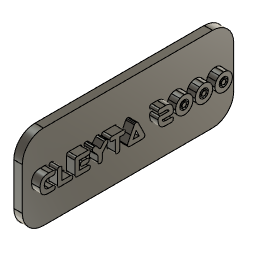
cleyta - placa v2 (Autodesk Fusion 360 design; units mm, degrees)
Autodesk Fusion 360 part; units mm, degrees
note: some values were not read from the file. Chosen so that the rebuilt part matches the saved one: which face or edge a step refers to.
(part 1 of 2)
sketch "Sketch1" plane through (0, 0, 0) normal (1, 0, 0) x (0, 1, 0)
  line L0 (-62.7452, 16.4403) -> (-22.7452, 16.4403)
  line L1 (-17.7452, 11.4403) -> (-17.7452, 1.4403)
  line L2 (-22.7452, -3.5597) -> (-62.7452, -3.5597)
  line L3 (-67.7452, 1.4403) -> (-67.7452, 11.4403)
  arc A0 (-62.7452, 16.4403) -> (-67.7452, 11.4403) centre (-62.7452, 11.4403) ccw
  arc A1 (-17.7452, 11.4403) -> (-22.7452, 16.4403) centre (-22.7452, 11.4403) ccw
  arc A2 (-22.7452, -3.5597) -> (-17.7452, 1.4403) centre (-22.7452, 1.4403) ccw
  arc A3 (-67.7452, 1.4403) -> (-62.7452, -3.5597) centre (-62.7452, 1.4403) ccw
  point P0 (-67.7452, 16.4403)
  point P1 (-17.7452, 16.4403)
  point P2 (-67.7452, -3.5597)
  dimension "d1" = 50
  dimension "d2" = 20
  dimension "d3" = 5
  constraint horizontal L0
  constraint vertical L1
  constraint horizontal L2
  constraint vertical L3
  constraint coincident P0 L0
  constraint coincident P0 L3
  constraint tangent L0 A0
  constraint tangent L3 A0
  constraint coincident P1 L0
  constraint coincident P1 L1
  constraint tangent L0 A1
  constraint tangent L1 A1
  constraint equal A0 A1
  constraint tangent L1 A2
  constraint tangent L2 A2
  constraint equal A0 A2
  constraint coincident P2 L2
  constraint coincident P2 L3
  constraint tangent L2 A3
  constraint tangent L3 A3
  constraint equal A0 A3
  measures "d1" distance of P0 P1
  measures "d2" distance of P0 P2
  measures "d3" radius of A0
extrude "Extrude1" add sketch "Sketch1" along normal blind 5
sketch "Sketch2" plane through (5, 0, 0) normal (1, 0, 0) x (0, 1, 0)
  arc A0 (-62.7452, 16.4403) -> (-67.7452, 11.4403) centre (-62.7452, 11.4403) ccw
  line L0 (-67.7452, 11.4403) -> (-67.7452, 1.4403)
  arc A1 (-67.7452, 1.4403) -> (-62.7452, -3.5597) centre (-62.7452, 1.4403) ccw
  line L1 (-62.7452, -3.5597) -> (-22.7452, -3.5597)
  arc A2 (-22.7452, -3.5597) -> (-17.7452, 1.4403) centre (-22.7452, 1.4403) ccw
  line L2 (-17.7452, 1.4403) -> (-17.7452, 11.4403)
  arc A3 (-17.7452, 11.4403) -> (-22.7452, 16.4403) centre (-22.7452, 11.4403) ccw
  line L3 (-22.7452, 16.4403) -> (-62.7452, 16.4403)
  line L4 (-62.4235, 8.5936) -> (-61.4376, 8.5911)
  spline S0 degree 3 poles (-61.4376, 8.5911) (-61.1111, 8.5861) (-60.9466, 8.4234) (-60.9447, 8.1031) knots 0 0 0 0 1 1 1 1
  spline S1 degree 3 poles (-60.9447, 8.1031) (-60.9466, 7.771) (-61.1117, 7.6058) (-61.4401, 7.6077) knots 0 0 0 0 1 1 1 1
  line L5 (-61.4401, 7.6077) -> (-62.421, 7.6052)
  spline S2 degree 3 poles (-62.421, 7.6052) (-63.0766, 7.6102) (-63.4044, 7.283) (-63.4044, 6.6243) knots 0 0 0 0 1 1 1 1
  spline S3 degree 3 poles (-63.4044, 6.6243) (-63.4044, 5.97) (-63.0766, 5.6415) (-62.421, 5.6384) knots 0 0 0 0 1 1 1 1
  line L6 (-62.421, 5.6384) -> (-61.4401, 5.6384)
  spline S4 degree 3 poles (-61.4401, 5.6384) (-61.1117, 5.6315) (-60.9472, 5.4689) (-60.9472, 5.1505) knots 0 0 0 0 1 1 1 1
  spline S5 degree 3 poles (-60.9472, 5.1505) (-60.9472, 4.8214) (-61.1098, 4.6563) (-61.4351, 4.655) knots 0 0 0 0 1 1 1 1
  line L7 (-61.4351, 4.655) -> (-62.421, 4.655)
  spline S6 degree 3 poles (-62.421, 4.655) (-63.7341, 4.655) (-64.3915, 5.3119) (-64.3928, 6.6268) knots 0 0 0 0 1 1 1 1
  spline S7 degree 3 poles (-64.3928, 6.6268) (-64.3928, 7.9392) (-63.7366, 8.5948) (-62.4235, 8.5936) knots 0 0 0 0 1 1 1 1
  spline S8 degree 3 poles (-59.9613, 8.5986) (-59.631, 8.5898) (-59.4646, 8.4291) (-59.4608, 8.1157) knots 0 0 0 0 1 1 1 1
  line L8 (-59.4608, 8.1157) -> (-59.4658, 5.6434)
  line L9 (-59.4658, 5.6434) -> (-57.509, 5.6434)
  spline S9 degree 3 poles (-57.509, 5.6434) (-57.1775, 5.6415) (-57.0111, 5.4758) (-57.0111, 5.1455) knots 0 0 0 0 1 1 1 1
  spline S10 degree 3 poles (-57.0111, 5.1455) (-57.013, 4.8214) (-57.1756, 4.6582) (-57.499, 4.655) knots 0 0 0 0 1 1 1 1
  line L10 (-57.499, 4.655) -> (-59.9613, 4.655)
  spline S11 degree 3 poles (-59.9613, 4.655) (-60.2884, 4.655) (-60.4529, 4.8139) (-60.4542, 5.133) knots 0 0 0 0 1 1 1 1
  line L11 (-60.4542, 5.133) -> (-60.4542, 8.1006)
  spline S12 degree 3 poles (-60.4542, 8.1006) (-60.4529, 8.4259) (-60.2884, 8.5917) (-59.9613, 8.5986) knots 0 0 0 0 1 1 1 1
  line L12 (-56.0227, 8.5986) -> (-53.5304, 8.5936)
  spline S13 degree 3 poles (-53.5304, 8.5936) (-53.2239, 8.5886) (-53.0694, 8.4291) (-53.0675, 8.1157) knots 0 0 0 0 1 1 1 1
  spline S14 degree 3 poles (-53.0675, 8.1157) (-53.0675, 7.7804) (-53.2339, 7.6102) (-53.5654, 7.6052) knots 0 0 0 0 1 1 1 1
  line L13 (-53.5654, 7.6052) -> (-55.5272, 7.6052)
  line L14 (-55.5272, 7.6052) -> (-55.5272, 5.6434)
  line L15 (-55.5272, 5.6434) -> (-53.5704, 5.6434)
  spline S15 degree 3 poles (-53.5704, 5.6434) (-53.2389, 5.6415) (-53.0725, 5.4758) (-53.0725, 5.1455) knots 0 0 0 0 1 1 1 1
  spline S16 degree 3 poles (-53.0725, 5.1455) (-53.0744, 4.8214) (-53.237, 4.6582) (-53.5604, 4.655) knots 0 0 0 0 1 1 1 1
  line L16 (-53.5604, 4.655) -> (-56.0227, 4.655)
  spline S17 degree 3 poles (-56.0227, 4.655) (-56.3498, 4.655) (-56.5144, 4.8139) (-56.5156, 5.133) knots 0 0 0 0 1 1 1 1
  line L17 (-56.5156, 5.133) -> (-56.5156, 8.1006)
  spline S18 degree 3 poles (-56.5156, 8.1006) (-56.5144, 8.4259) (-56.3498, 8.5917) (-56.0227, 8.5986) knots 0 0 0 0 1 1 1 1
  spline S19 degree 3 poles (-55.292, 6.6143) (-55.2889, 6.9408) (-55.1262, 7.1072) (-54.8041, 7.1122) knots 0 0 0 0 1 1 1 1
  line L18 (-54.8041, 7.1122) -> (-53.8132, 7.1122)
  spline S20 degree 3 poles (-53.8132, 7.1122) (-53.4847, 7.1085) (-53.3177, 6.9446) (-53.3127, 6.6193) knots 0 0 0 0 1 1 1 1
  spline S21 degree 3 poles (-53.3127, 6.6193) (-53.3196, 6.2903) (-53.4854, 6.1264) (-53.8107, 6.1264) knots 0 0 0 0 1 1 1 1
  line L19 (-53.8107, 6.1264) -> (-54.8016, 6.1264)
  spline S22 degree 3 poles (-54.8016, 6.1264) (-55.1268, 6.1245) (-55.2907, 6.2871) (-55.292, 6.6143) knots 0 0 0 0 1 1 1 1
  spline S23 degree 3 poles (-52.0766, 8.6036) (-51.9133, 8.6036) (-51.79, 8.5623) (-51.7062, 8.481) knots 0 0 0 0 1 1 1 1
  spline S24 degree 3 poles (-51.7062, 8.481) (-51.623, 8.4009) (-51.3309, 8.0581) (-50.8304, 7.4526) knots 0 0 0 0 1 1 1 1
  spline S25 degree 3 poles (-50.8304, 7.4526) (-50.3218, 8.0681) (-50.026, 8.4159) (-49.9421, 8.496) knots 0 0 0 0 1 1 1 1
  spline S26 degree 3 poles (-49.9421, 8.496) (-49.8589, 8.5761) (-49.7357, 8.6161) (-49.5718, 8.6161) knots 0 0 0 0 1 1 1 1
  spline S27 degree 3 poles (-49.5718, 8.6161) (-49.4116, 8.6161) (-49.2884, 8.5742) (-49.2015, 8.491) knots 0 0 0 0 1 1 1 1
  spline S28 degree 3 poles (-49.2015, 8.491) (-49.1151, 8.4072) (-49.0738, 8.2833) (-49.0788, 8.1182) knots 0 0 0 0 1 1 1 1
  spline S29 degree 3 poles (-49.0788, 8.1182) (-49.0788, 7.9442) (-49.1658, 7.7816) (-49.3391, 7.6302) knots 0 0 0 0 1 1 1 1
  line L20 (-49.3391, 7.6302) -> (-50.3475, 6.4542)
  line L21 (-50.3475, 6.4542) -> (-50.35, 5.1455)
  spline S30 degree 3 poles (-50.35, 5.1455) (-50.3569, 4.8233) (-50.522, 4.66) (-50.8454, 4.655) knots 0 0 0 0 1 1 1 1
  spline S31 degree 3 poles (-50.8454, 4.655) (-51.1707, 4.6469) (-51.3334, 4.8152) (-51.3334, 5.1605) knots 0 0 0 0 1 1 1 1
  line L22 (-51.3334, 5.1605) -> (-51.3384, 6.4592)
  line L23 (-51.3384, 6.4592) -> (-52.3093, 7.6152)
  spline S32 degree 3 poles (-52.3093, 7.6152) (-52.4832, 7.7685) (-52.5695, 7.9317) (-52.5695, 8.1056) knots 0 0 0 0 1 1 1 1
  spline S33 degree 3 poles (-52.5695, 8.1056) (-52.5745, 8.272) (-52.5345, 8.3965) (-52.4494, 8.4785) knots 0 0 0 0 1 1 1 1
  spline S34 degree 3 poles (-52.4494, 8.4785) (-52.3631, 8.5617) (-52.2386, 8.6036) (-52.0766, 8.6036) knots 0 0 0 0 1 1 1 1
  line L24 (-48.1405, 8.5986) -> (-45.6483, 8.5936)
  spline S35 degree 3 poles (-45.6483, 8.5936) (-45.3418, 8.5886) (-45.1872, 8.4291) (-45.1854, 8.1157) knots 0 0 0 0 1 1 1 1
  spline S36 degree 3 poles (-45.1854, 8.1157) (-45.1854, 7.7804) (-45.3518, 7.6102) (-45.6833, 7.6052) knots 0 0 0 0 1 1 1 1
  line L25 (-45.6833, 7.6052) -> (-46.419, 7.6052)
  line L26 (-46.419, 7.6052) -> (-46.4165, 5.1455)
  spline S37 degree 3 poles (-46.4165, 5.1455) (-46.4202, 4.8214) (-46.5854, 4.6582) (-46.9119, 4.655) knots 0 0 0 0 1 1 1 1
  spline S38 degree 3 poles (-46.9119, 4.655) (-47.241, 4.655) (-47.4049, 4.8139) (-47.4049, 5.133) knots 0 0 0 0 1 1 1 1
  line L27 (-47.4049, 5.133) -> (-47.4024, 7.6052)
  line L28 (-47.4024, 7.6052) -> (-48.1405, 7.6052)
  spline S39 degree 3 poles (-48.1405, 7.6052) (-48.4696, 7.6052) (-48.6335, 7.7703) (-48.6335, 8.1006) knots 0 0 0 0 1 1 1 1
  spline S40 degree 3 poles (-48.6335, 8.1006) (-48.6322, 8.4259) (-48.4677, 8.5917) (-48.1405, 8.5986) knots 0 0 0 0 1 1 1 1
  spline S41 degree 3 poles (-44.1994, 4.6525) (-44.2833, 4.6525) (-44.364, 4.6732) (-44.4422, 4.7151) knots 0 0 0 0 1 1 1 1
  spline S42 degree 3 poles (-44.4422, 4.7151) (-44.521, 4.7564) (-44.5823, 4.8164) (-44.6273, 4.8952) knots 0 0 0 0 1 1 1 1
  spline S43 degree 3 poles (-44.6273, 4.8952) (-44.6711, 4.9753) (-44.6924, 5.0585) (-44.6924, 5.1455) knots 0 0 0 0 1 1 1 1
  spline S44 degree 3 poles (-44.6924, 5.1455) (-44.6924, 5.2305) (-44.4472, 5.766) (-43.9567, 6.7519) knots 0 0 0 0 1 1 1 1
  spline S45 degree 3 poles (-43.9567, 6.7519) (-43.465, 7.7391) (-43.1979, 8.272) (-43.156, 8.3509) knots 0 0 0 0 1 1 1 1
  spline S46 degree 3 poles (-43.156, 8.3509) (-43.1128, 8.4291) (-43.0522, 8.4897) (-42.9733, 8.5335) knots 0 0 0 0 1 1 1 1
  spline S47 degree 3 poles (-42.9733, 8.5335) (-42.8951, 8.5767) (-42.8126, 8.5986) (-42.7256, 8.5986) knots 0 0 0 0 1 1 1 1
  spline S48 degree 3 poles (-42.7256, 8.5986) (-42.6405, 8.5986) (-42.5598, 8.5767) (-42.4829, 8.5335) knots 0 0 0 0 1 1 1 1
  spline S49 degree 3 poles (-42.4829, 8.5335) (-42.4047, 8.4897) (-42.344, 8.4291) (-42.3002, 8.3509) knots 0 0 0 0 1 1 1 1
  spline S50 degree 3 poles (-42.3002, 8.3509) (-42.2571, 8.272) (-41.9887, 7.7391) (-41.4945, 6.7519) knots 0 0 0 0 1 1 1 1
  spline S51 degree 3 poles (-41.4945, 6.7519) (-41.0009, 5.766) (-40.7538, 5.2305) (-40.7538, 5.1455) knots 0 0 0 0 1 1 1 1
  spline S52 degree 3 poles (-40.7538, 5.1455) (-40.7538, 5.0585) (-40.7763, 4.9753) (-40.8214, 4.8952) knots 0 0 0 0 1 1 1 1
  spline S53 degree 3 poles (-40.8214, 4.8952) (-40.8652, 4.8164) (-40.9265, 4.7564) (-41.0066, 4.7151) knots 0 0 0 0 1 1 1 1
  spline S54 degree 3 poles (-41.0066, 4.7151) (-41.0854, 4.6732) (-41.1654, 4.6525) (-41.2468, 4.6525) knots 0 0 0 0 1 1 1 1
  line L29 (-41.2468, 4.6525) -> (-44.1994, 4.6525)
  line L30 (-42.0525, 5.6459) -> (-42.7256, 7.0322)
  line L31 (-42.7256, 7.0322) -> (-43.4037, 5.6459)
  line L32 (-43.4037, 5.6459) -> (-42.0525, 5.6459)
  spline S55 degree 3 poles (-36.0764, 8.5936) (-34.9272, 8.5948) (-34.3517, 7.9386) (-34.3498, 6.6243) knots 0 0 0 0 1 1 1 1
  spline S56 degree 3 poles (-34.3498, 6.6243) (-34.3486, 6.2953) (-34.5125, 6.132) (-34.8428, 6.1339) knots 0 0 0 0 1 1 1 1
  line L33 (-34.8428, 6.1339) -> (-36.8146, 6.1364)
  spline S57 degree 3 poles (-36.8146, 6.1364) (-36.8114, 5.8061) (-36.5662, 5.6397) (-36.0789, 5.6384) knots 0 0 0 0 1 1 1 1
  line L34 (-36.0789, 5.6384) -> (-34.8403, 5.6434)
  spline S58 degree 3 poles (-34.8403, 5.6434) (-34.5187, 5.6415) (-34.3548, 5.4764) (-34.3498, 5.148) knots 0 0 0 0 1 1 1 1
  spline S59 degree 3 poles (-34.3498, 5.148) (-34.3517, 4.8177) (-34.5162, 4.6538) (-34.8428, 4.655) knots 0 0 0 0 1 1 1 1
  line L35 (-34.8428, 4.655) -> (-36.0714, 4.655)
  spline S60 degree 3 poles (-36.0714, 4.655) (-37.2243, 4.6563) (-37.8017, 5.3137) (-37.803, 6.6268) knots 0 0 0 0 1 1 1 1
  spline S61 degree 3 poles (-37.803, 6.6268) (-37.8017, 6.9521) (-37.6372, 7.1154) (-37.31, 7.1173) knots 0 0 0 0 1 1 1 1
  line L36 (-37.31, 7.1173) -> (-35.3382, 7.1147)
  spline S62 degree 3 poles (-35.3382, 7.1147) (-35.3382, 7.4432) (-35.5809, 7.6064) (-36.0664, 7.6052) knots 0 0 0 0 1 1 1 1
  line L37 (-36.0664, 7.6052) -> (-37.305, 7.6052)
  spline S63 degree 3 poles (-37.305, 7.6052) (-37.6303, 7.6133) (-37.7967, 7.7791) (-37.803, 8.1031) knots 0 0 0 0 1 1 1 1
  spline S64 degree 3 poles (-37.803, 8.1031) (-37.7948, 8.4316) (-37.629, 8.5948) (-37.305, 8.5936) knots 0 0 0 0 1 1 1 1
  line L38 (-37.305, 8.5936) -> (-36.0764, 8.5936)
  spline S65 degree 3 poles (-31.8926, 8.5936) (-31.5623, 8.5936) (-31.2408, 8.5085) (-30.9267, 8.3384) knots 0 0 0 0 1 1 1 1
  spline S66 degree 3 poles (-30.9267, 8.3384) (-30.6115, 8.1682) (-30.365, 7.9242) (-30.1861, 7.6077) knots 0 0 0 0 1 1 1 1
  spline S67 degree 3 poles (-30.1861, 7.6077) (-30.0078, 7.2924) (-29.9183, 6.9634) (-29.9183, 6.6218) knots 0 0 0 0 1 1 1 1
  spline S68 degree 3 poles (-29.9183, 6.6218) (-29.9183, 6.2796) (-30.0053, 5.9518) (-30.1786, 5.6384) knots 0 0 0 0 1 1 1 1
  spline S69 degree 3 poles (-30.1786, 5.6384) (-30.3525, 5.3263) (-30.5958, 5.0835) (-30.9092, 4.9103) knots 0 0 0 0 1 1 1 1
  spline S70 degree 3 poles (-30.9092, 4.9103) (-31.2233, 4.7363) (-31.5511, 4.65) (-31.8926, 4.65) knots 0 0 0 0 1 1 1 1
  spline S71 degree 3 poles (-31.8926, 4.65) (-32.2329, 4.65) (-32.5601, 4.7363) (-32.8735, 4.9103) knots 0 0 0 0 1 1 1 1
  spline S72 degree 3 poles (-32.8735, 4.9103) (-33.1875, 5.0835) (-33.4309, 5.3263) (-33.6042, 5.6384) knots 0 0 0 0 1 1 1 1
  spline S73 degree 3 poles (-33.6042, 5.6384) (-33.7781, 5.9518) (-33.8644, 6.2796) (-33.8644, 6.6218) knots 0 0 0 0 1 1 1 1
  spline S74 degree 3 poles (-33.8644, 6.6218) (-33.8644, 6.9634) (-33.7768, 7.2924) (-33.6017, 7.6077) knots 0 0 0 0 1 1 1 1
  spline S75 degree 3 poles (-33.6017, 7.6077) (-33.4253, 7.9242) (-33.18, 8.1682) (-32.866, 8.3384) knots 0 0 0 0 1 1 1 1
  spline S76 degree 3 poles (-32.866, 8.3384) (-32.5507, 8.5085) (-32.2267, 8.5936) (-31.8926, 8.5936) knots 0 0 0 0 1 1 1 1
  spline S77 degree 3 poles (-31.8901, 7.6127) (-32.0571, 7.6127) (-32.2192, 7.5702) (-32.3756, 7.4851) knots 0 0 0 0 1 1 1 1
  spline S78 degree 3 poles (-32.3756, 7.4851) (-32.5326, 7.4013) (-32.6552, 7.2805) (-32.7434, 7.1223) knots 0 0 0 0 1 1 1 1
  spline S79 degree 3 poles (-32.7434, 7.1223) (-32.8322, 6.9634) (-32.876, 6.7982) (-32.876, 6.6268) knots 0 0 0 0 1 1 1 1
  spline S80 degree 3 poles (-32.876, 6.6268) (-32.876, 6.4548) (-32.8328, 6.2903) (-32.7459, 6.1339) knots 0 0 0 0 1 1 1 1
  spline S81 degree 3 poles (-32.7459, 6.1339) (-32.6596, 5.9787) (-32.5376, 5.8574) (-32.3806, 5.771) knots 0 0 0 0 1 1 1 1
  spline S82 degree 3 poles (-32.3806, 5.771) (-32.2242, 5.6841) (-32.0603, 5.6409) (-31.8901, 5.6409) knots 0 0 0 0 1 1 1 1
  spline S83 degree 3 poles (-31.8901, 5.6409) (-31.7187, 5.6409) (-31.5542, 5.6841) (-31.3972, 5.771) knots 0 0 0 0 1 1 1 1
  spline S84 degree 3 poles (-31.3972, 5.771) (-31.2408, 5.8574) (-31.1188, 5.9787) (-31.0318, 6.1339) knots 0 0 0 0 1 1 1 1
  spline S85 degree 3 poles (-31.0318, 6.1339) (-30.9455, 6.2903) (-30.9017, 6.4548) (-30.9017, 6.6268) knots 0 0 0 0 1 1 1 1
  spline S86 degree 3 poles (-30.9017, 6.6268) (-30.9017, 6.7982) (-30.9461, 6.9634) (-31.0343, 7.1223) knots 0 0 0 0 1 1 1 1
  spline S87 degree 3 poles (-31.0343, 7.1223) (-31.1232, 7.2805) (-31.2464, 7.4013) (-31.4047, 7.4851) knots 0 0 0 0 1 1 1 1
  spline S88 degree 3 poles (-31.4047, 7.4851) (-31.5617, 7.5702) (-31.7237, 7.6127) (-31.8901, 7.6127) knots 0 0 0 0 1 1 1 1
  spline S89 degree 3 poles (-31.8926, 7.1072) (-31.8113, 7.1072) (-31.7318, 7.0853) (-31.6549, 7.0422) knots 0 0 0 0 1 1 1 1
  spline S90 degree 3 poles (-31.6549, 7.0422) (-31.5767, 7.0003) (-31.516, 6.9402) (-31.4722, 6.862) knots 0 0 0 0 1 1 1 1
  spline S91 degree 3 poles (-31.4722, 6.862) (-31.4272, 6.7851) (-31.4047, 6.7031) (-31.4047, 6.6168) knots 0 0 0 0 1 1 1 1
  spline S92 degree 3 poles (-31.4047, 6.6168) (-31.4047, 6.5317) (-31.4266, 6.4498) (-31.4697, 6.3716) knots 0 0 0 0 1 1 1 1
  spline S93 degree 3 poles (-31.4697, 6.3716) (-31.5135, 6.2946) (-31.5736, 6.2346) (-31.6499, 6.1914) knots 0 0 0 0 1 1 1 1
  spline S94 degree 3 poles (-31.6499, 6.1914) (-31.7268, 6.1495) (-31.8075, 6.1289) (-31.8926, 6.1289) knots 0 0 0 0 1 1 1 1
  spline S95 degree 3 poles (-31.8926, 6.1289) (-31.9796, 6.1289) (-32.0621, 6.1495) (-32.1403, 6.1914) knots 0 0 0 0 1 1 1 1
  spline S96 degree 3 poles (-32.1403, 6.1914) (-32.2173, 6.2346) (-32.2773, 6.2946) (-32.3205, 6.3716) knots 0 0 0 0 1 1 1 1
  spline S97 degree 3 poles (-32.3205, 6.3716) (-32.3624, 6.4498) (-32.3831, 6.5317) (-32.3831, 6.6168) knots 0 0 0 0 1 1 1 1
  spline S98 degree 3 poles (-32.3831, 6.6168) (-32.3831, 6.7031) (-32.3618, 6.7851) (-32.318, 6.862) knots 0 0 0 0 1 1 1 1
  spline S99 degree 3 poles (-32.318, 6.862) (-32.2748, 6.9402) (-32.2148, 7.0003) (-32.1378, 7.0422) knots 0 0 0 0 1 1 1 1
  spline S100 degree 3 poles (-32.1378, 7.0422) (-32.0596, 7.0853) (-31.9777, 7.1072) (-31.8926, 7.1072) knots 0 0 0 0 1 1 1 1
  spline S101 degree 3 poles (-27.4565, 8.5936) (-27.1262, 8.5936) (-26.8046, 8.5085) (-26.4906, 8.3384) knots 0 0 0 0 1 1 1 1
  spline S102 degree 3 poles (-26.4906, 8.3384) (-26.1753, 8.1682) (-25.9288, 7.9242) (-25.7499, 7.6077) knots 0 0 0 0 1 1 1 1
  spline S103 degree 3 poles (-25.7499, 7.6077) (-25.5716, 7.2924) (-25.4822, 6.9634) (-25.4822, 6.6218) knots 0 0 0 0 1 1 1 1
  spline S104 degree 3 poles (-25.4822, 6.6218) (-25.4822, 6.2796) (-25.5691, 5.9518) (-25.7424, 5.6384) knots 0 0 0 0 1 1 1 1
  spline S105 degree 3 poles (-25.7424, 5.6384) (-25.9163, 5.3263) (-26.1597, 5.0835) (-26.4731, 4.9103) knots 0 0 0 0 1 1 1 1
  spline S106 degree 3 poles (-26.4731, 4.9103) (-26.7871, 4.7363) (-27.1149, 4.65) (-27.4565, 4.65) knots 0 0 0 0 1 1 1 1
  spline S107 degree 3 poles (-27.4565, 4.65) (-27.7968, 4.65) (-28.1239, 4.7363) (-28.4373, 4.9103) knots 0 0 0 0 1 1 1 1
  spline S108 degree 3 poles (-28.4373, 4.9103) (-28.7514, 5.0835) (-28.9947, 5.3263) (-29.168, 5.6384) knots 0 0 0 0 1 1 1 1
  spline S109 degree 3 poles (-29.168, 5.6384) (-29.3419, 5.9518) (-29.4282, 6.2796) (-29.4282, 6.6218) knots 0 0 0 0 1 1 1 1
  spline S110 degree 3 poles (-29.4282, 6.6218) (-29.4282, 6.9634) (-29.3407, 7.2924) (-29.1655, 7.6077) knots 0 0 0 0 1 1 1 1
  spline S111 degree 3 poles (-29.1655, 7.6077) (-28.9891, 7.9242) (-28.7439, 8.1682) (-28.4298, 8.3384) knots 0 0 0 0 1 1 1 1
  spline S112 degree 3 poles (-28.4298, 8.3384) (-28.1146, 8.5085) (-27.7905, 8.5936) (-27.4565, 8.5936) knots 0 0 0 0 1 1 1 1
  spline S113 degree 3 poles (-27.454, 7.6127) (-27.621, 7.6127) (-27.783, 7.5702) (-27.9394, 7.4851) knots 0 0 0 0 1 1 1 1
  spline S114 degree 3 poles (-27.9394, 7.4851) (-28.0964, 7.4013) (-28.219, 7.2805) (-28.3072, 7.1223) knots 0 0 0 0 1 1 1 1
  spline S115 degree 3 poles (-28.3072, 7.1223) (-28.3961, 6.9634) (-28.4398, 6.7982) (-28.4398, 6.6268) knots 0 0 0 0 1 1 1 1
  spline S116 degree 3 poles (-28.4398, 6.6268) (-28.4398, 6.4548) (-28.3967, 6.2903) (-28.3097, 6.1339) knots 0 0 0 0 1 1 1 1
  spline S117 degree 3 poles (-28.3097, 6.1339) (-28.2234, 5.9787) (-28.1014, 5.8574) (-27.9444, 5.771) knots 0 0 0 0 1 1 1 1
  spline S118 degree 3 poles (-27.9444, 5.771) (-27.788, 5.6841) (-27.6241, 5.6409) (-27.454, 5.6409) knots 0 0 0 0 1 1 1 1
  spline S119 degree 3 poles (-27.454, 5.6409) (-27.2826, 5.6409) (-27.118, 5.6841) (-26.961, 5.771) knots 0 0 0 0 1 1 1 1
  spline S120 degree 3 poles (-26.961, 5.771) (-26.8046, 5.8574) (-26.6826, 5.9787) (-26.5957, 6.1339) knots 0 0 0 0 1 1 1 1
  spline S121 degree 3 poles (-26.5957, 6.1339) (-26.5094, 6.2903) (-26.4656, 6.4548) (-26.4656, 6.6268) knots 0 0 0 0 1 1 1 1
  spline S122 degree 3 poles (-26.4656, 6.6268) (-26.4656, 6.7982) (-26.51, 6.9634) (-26.5982, 7.1223) knots 0 0 0 0 1 1 1 1
  spline S123 degree 3 poles (-26.5982, 7.1223) (-26.687, 7.2805) (-26.8103, 7.4013) (-26.9685, 7.4851) knots 0 0 0 0 1 1 1 1
  spline S124 degree 3 poles (-26.9685, 7.4851) (-27.1255, 7.5702) (-27.2876, 7.6127) (-27.454, 7.6127) knots 0 0 0 0 1 1 1 1
  spline S125 degree 3 poles (-27.4565, 7.1072) (-27.3751, 7.1072) (-27.2957, 7.0853) (-27.2187, 7.0422) knots 0 0 0 0 1 1 1 1
  spline S126 degree 3 poles (-27.2187, 7.0422) (-27.1406, 7.0003) (-27.0799, 6.9402) (-27.0361, 6.862) knots 0 0 0 0 1 1 1 1
  spline S127 degree 3 poles (-27.0361, 6.862) (-26.991, 6.7851) (-26.9685, 6.7031) (-26.9685, 6.6168) knots 0 0 0 0 1 1 1 1
  spline S128 degree 3 poles (-26.9685, 6.6168) (-26.9685, 6.5317) (-26.9904, 6.4498) (-27.0336, 6.3716) knots 0 0 0 0 1 1 1 1
  spline S129 degree 3 poles (-27.0336, 6.3716) (-27.0774, 6.2946) (-27.1374, 6.2346) (-27.2137, 6.1914) knots 0 0 0 0 1 1 1 1
  spline S130 degree 3 poles (-27.2137, 6.1914) (-27.2907, 6.1495) (-27.3714, 6.1289) (-27.4565, 6.1289) knots 0 0 0 0 1 1 1 1
  spline S131 degree 3 poles (-27.4565, 6.1289) (-27.5434, 6.1289) (-27.626, 6.1495) (-27.7042, 6.1914) knots 0 0 0 0 1 1 1 1
  spline S132 degree 3 poles (-27.7042, 6.1914) (-27.7811, 6.2346) (-27.8412, 6.2946) (-27.8843, 6.3716) knots 0 0 0 0 1 1 1 1
  spline S133 degree 3 poles (-27.8843, 6.3716) (-27.9263, 6.4498) (-27.9469, 6.5317) (-27.9469, 6.6168) knots 0 0 0 0 1 1 1 1
  spline S134 degree 3 poles (-27.9469, 6.6168) (-27.9469, 6.7031) (-27.9256, 6.7851) (-27.8818, 6.862) knots 0 0 0 0 1 1 1 1
  spline S135 degree 3 poles (-27.8818, 6.862) (-27.8387, 6.9402) (-27.7786, 7.0003) (-27.7017, 7.0422) knots 0 0 0 0 1 1 1 1
  spline S136 degree 3 poles (-27.7017, 7.0422) (-27.6235, 7.0853) (-27.5415, 7.1072) (-27.4565, 7.1072) knots 0 0 0 0 1 1 1 1
  spline S137 degree 3 poles (-23.0203, 8.5936) (-22.69, 8.5936) (-22.3685, 8.5085) (-22.0544, 8.3384) knots 0 0 0 0 1 1 1 1
  spline S138 degree 3 poles (-22.0544, 8.3384) (-21.7391, 8.1682) (-21.4927, 7.9242) (-21.3138, 7.6077) knots 0 0 0 0 1 1 1 1
  spline S139 degree 3 poles (-21.3138, 7.6077) (-21.1355, 7.2924) (-21.046, 6.9634) (-21.046, 6.6218) knots 0 0 0 0 1 1 1 1
  spline S140 degree 3 poles (-21.046, 6.6218) (-21.046, 6.2796) (-21.133, 5.9518) (-21.3063, 5.6384) knots 0 0 0 0 1 1 1 1
  spline S141 degree 3 poles (-21.3063, 5.6384) (-21.4802, 5.3263) (-21.7235, 5.0835) (-22.0369, 4.9103) knots 0 0 0 0 1 1 1 1
  spline S142 degree 3 poles (-22.0369, 4.9103) (-22.3509, 4.7363) (-22.6787, 4.65) (-23.0203, 4.65) knots 0 0 0 0 1 1 1 1
  spline S143 degree 3 poles (-23.0203, 4.65) (-23.3606, 4.65) (-23.6878, 4.7363) (-24.0012, 4.9103) knots 0 0 0 0 1 1 1 1
  spline S144 degree 3 poles (-24.0012, 4.9103) (-24.3152, 5.0835) (-24.5586, 5.3263) (-24.7319, 5.6384) knots 0 0 0 0 1 1 1 1
  spline S145 degree 3 poles (-24.7319, 5.6384) (-24.9058, 5.9518) (-24.9921, 6.2796) (-24.9921, 6.6218) knots 0 0 0 0 1 1 1 1
  spline S146 degree 3 poles (-24.9921, 6.6218) (-24.9921, 6.9634) (-24.9045, 7.2924) (-24.7293, 7.6077) knots 0 0 0 0 1 1 1 1
  spline S147 degree 3 poles (-24.7293, 7.6077) (-24.5529, 7.9242) (-24.3077, 8.1682) (-23.9937, 8.3384) knots 0 0 0 0 1 1 1 1
  spline S148 degree 3 poles (-23.9937, 8.3384) (-23.6784, 8.5085) (-23.3544, 8.5936) (-23.0203, 8.5936) knots 0 0 0 0 1 1 1 1
  spline S149 degree 3 poles (-23.0178, 7.6127) (-23.1848, 7.6127) (-23.3468, 7.5702) (-23.5032, 7.4851) knots 0 0 0 0 1 1 1 1
  spline S150 degree 3 poles (-23.5032, 7.4851) (-23.6603, 7.4013) (-23.7829, 7.2805) (-23.8711, 7.1223) knots 0 0 0 0 1 1 1 1
  spline S151 degree 3 poles (-23.8711, 7.1223) (-23.9599, 6.9634) (-24.0037, 6.7982) (-24.0037, 6.6268) knots 0 0 0 0 1 1 1 1
  spline S152 degree 3 poles (-24.0037, 6.6268) (-24.0037, 6.4548) (-23.9605, 6.2903) (-23.8736, 6.1339) knots 0 0 0 0 1 1 1 1
  spline S153 degree 3 poles (-23.8736, 6.1339) (-23.7872, 5.9787) (-23.6653, 5.8574) (-23.5082, 5.771) knots 0 0 0 0 1 1 1 1
  spline S154 degree 3 poles (-23.5082, 5.771) (-23.3519, 5.6841) (-23.188, 5.6409) (-23.0178, 5.6409) knots 0 0 0 0 1 1 1 1
  spline S155 degree 3 poles (-23.0178, 5.6409) (-22.8464, 5.6409) (-22.6819, 5.6841) (-22.5249, 5.771) knots 0 0 0 0 1 1 1 1
  spline S156 degree 3 poles (-22.5249, 5.771) (-22.3685, 5.8574) (-22.2465, 5.9787) (-22.1595, 6.1339) knots 0 0 0 0 1 1 1 1
  spline S157 degree 3 poles (-22.1595, 6.1339) (-22.0732, 6.2903) (-22.0294, 6.4548) (-22.0294, 6.6268) knots 0 0 0 0 1 1 1 1
  spline S158 degree 3 poles (-22.0294, 6.6268) (-22.0294, 6.7982) (-22.0738, 6.9634) (-22.162, 7.1223) knots 0 0 0 0 1 1 1 1
  spline S159 degree 3 poles (-22.162, 7.1223) (-22.2509, 7.2805) (-22.3741, 7.4013) (-22.5324, 7.4851) knots 0 0 0 0 1 1 1 1
  spline S160 degree 3 poles (-22.5324, 7.4851) (-22.6894, 7.5702) (-22.8514, 7.6127) (-23.0178, 7.6127) knots 0 0 0 0 1 1 1 1
  spline S161 degree 3 poles (-23.0203, 7.1072) (-22.939, 7.1072) (-22.8595, 7.0853) (-22.7826, 7.0422) knots 0 0 0 0 1 1 1 1
  spline S162 degree 3 poles (-22.7826, 7.0422) (-22.7044, 7.0003) (-22.6437, 6.9402) (-22.5999, 6.862) knots 0 0 0 0 1 1 1 1
  spline S163 degree 3 poles (-22.5999, 6.862) (-22.5549, 6.7851) (-22.5324, 6.7031) (-22.5324, 6.6168) knots 0 0 0 0 1 1 1 1
  spline S164 degree 3 poles (-22.5324, 6.6168) (-22.5324, 6.5317) (-22.5543, 6.4498) (-22.5974, 6.3716) knots 0 0 0 0 1 1 1 1
  spline S165 degree 3 poles (-22.5974, 6.3716) (-22.6412, 6.2946) (-22.7013, 6.2346) (-22.7776, 6.1914) knots 0 0 0 0 1 1 1 1
  spline S166 degree 3 poles (-22.7776, 6.1914) (-22.8545, 6.1495) (-22.9352, 6.1289) (-23.0203, 6.1289) knots 0 0 0 0 1 1 1 1
  spline S167 degree 3 poles (-23.0203, 6.1289) (-23.1073, 6.1289) (-23.1898, 6.1495) (-23.268, 6.1914) knots 0 0 0 0 1 1 1 1
  spline S168 degree 3 poles (-23.268, 6.1914) (-23.345, 6.2346) (-23.405, 6.2946) (-23.4482, 6.3716) knots 0 0 0 0 1 1 1 1
  spline S169 degree 3 poles (-23.4482, 6.3716) (-23.4901, 6.4498) (-23.5107, 6.5317) (-23.5107, 6.6168) knots 0 0 0 0 1 1 1 1
  spline S170 degree 3 poles (-23.5107, 6.6168) (-23.5107, 6.7031) (-23.4895, 6.7851) (-23.4457, 6.862) knots 0 0 0 0 1 1 1 1
  spline S171 degree 3 poles (-23.4457, 6.862) (-23.4025, 6.9402) (-23.3425, 7.0003) (-23.2655, 7.0422) knots 0 0 0 0 1 1 1 1
  spline S172 degree 3 poles (-23.2655, 7.0422) (-23.1873, 7.0853) (-23.1054, 7.1072) (-23.0203, 7.1072) knots 0 0 0 0 1 1 1 1
extrude "Extrude4" cut 1 faces at (5, -36.0786, 3.1069) along direction (-1, 0, 0) blind 3
sketch "Sketch5" plane through (2, 0, 0) normal (1, 0, 0) x (0, 1, 0)
  arc A0 (-62.7452, 16.4403) -> (-67.7452, 11.4403) centre (-62.7452, 11.4403) ccw
  line L0 (-67.7452, 11.4403) -> (-67.7452, 1.4403)
  arc A1 (-67.7452, 1.4403) -> (-62.7452, -3.5597) centre (-62.7452, 1.4403) ccw
  line L1 (-62.7452, -3.5597) -> (-22.7452, -3.5597)
  arc A2 (-22.7452, -3.5597) -> (-17.7452, 1.4403) centre (-22.7452, 1.4403) ccw
  line L2 (-17.7452, 1.4403) -> (-17.7452, 11.4403)
  arc A3 (-17.7452, 11.4403) -> (-22.7452, 16.4403) centre (-22.7452, 11.4403) ccw
  line L3 (-22.7452, 16.4403) -> (-62.7452, 16.4403)
  line L4 (-63.4941, 8.6057) -> (-62.4588, 8.6031)
  spline S0 degree 3 poles (-62.4588, 8.6031) (-62.1159, 8.5978) (-61.9432, 8.427) (-61.9412, 8.0907) knots 0 0 0 0 1 1 1 1
  spline S1 degree 3 poles (-61.9412, 8.0907) (-61.9432, 7.7419) (-62.1166, 7.5685) (-62.4615, 7.5705) knots 0 0 0 0 1 1 1 1
  line L5 (-62.4615, 7.5705) -> (-63.4914, 7.5678)
  spline S2 degree 3 poles (-63.4914, 7.5678) (-64.1798, 7.5731) (-64.524, 7.2296) (-64.524, 6.5379) knots 0 0 0 0 1 1 1 1
  spline S3 degree 3 poles (-64.524, 6.5379) (-64.524, 5.8508) (-64.1798, 5.5059) (-63.4914, 5.5026) knots 0 0 0 0 1 1 1 1
  line L6 (-63.4914, 5.5026) -> (-62.4615, 5.5026)
  spline S4 degree 3 poles (-62.4615, 5.5026) (-62.1166, 5.4954) (-61.9438, 5.3246) (-61.9438, 4.9903) knots 0 0 0 0 1 1 1 1
  spline S5 degree 3 poles (-61.9438, 4.9903) (-61.9438, 4.6447) (-62.1146, 4.4713) (-62.4562, 4.47) knots 0 0 0 0 1 1 1 1
  line L7 (-62.4562, 4.47) -> (-63.4914, 4.47)
  spline S6 degree 3 poles (-63.4914, 4.47) (-64.8702, 4.47) (-65.5606, 5.1597) (-65.5619, 6.5405) knots 0 0 0 0 1 1 1 1
  spline S7 degree 3 poles (-65.5619, 6.5405) (-65.5619, 7.9186) (-64.8728, 8.607) (-63.4941, 8.6057) knots 0 0 0 0 1 1 1 1
  spline S8 degree 3 poles (-60.9086, 8.611) (-60.5617, 8.6018) (-60.387, 8.4329) (-60.3831, 8.1039) knots 0 0 0 0 1 1 1 1
  line L8 (-60.3831, 8.1039) -> (-60.3883, 5.5079)
  line L9 (-60.3883, 5.5079) -> (-58.3336, 5.5079)
  spline S9 degree 3 poles (-58.3336, 5.5079) (-57.9855, 5.5059) (-57.8107, 5.3318) (-57.8107, 4.985) knots 0 0 0 0 1 1 1 1
  spline S10 degree 3 poles (-57.8107, 4.985) (-57.8127, 4.6447) (-57.9835, 4.4733) (-58.3231, 4.47) knots 0 0 0 0 1 1 1 1
  line L10 (-58.3231, 4.47) -> (-60.9086, 4.47)
  spline S11 degree 3 poles (-60.9086, 4.47) (-61.2521, 4.47) (-61.4249, 4.6369) (-61.4262, 4.9719) knots 0 0 0 0 1 1 1 1
  line L11 (-61.4262, 4.9719) -> (-61.4262, 8.0881)
  spline S12 degree 3 poles (-61.4262, 8.0881) (-61.4249, 8.4297) (-61.2521, 8.6037) (-60.9086, 8.611) knots 0 0 0 0 1 1 1 1
  line L12 (-56.7728, 8.611) -> (-54.1558, 8.6057)
  spline S13 degree 3 poles (-54.1558, 8.6057) (-53.834, 8.6004) (-53.6717, 8.4329) (-53.6698, 8.1039) knots 0 0 0 0 1 1 1 1
  spline S14 degree 3 poles (-53.6698, 8.1039) (-53.6698, 7.7518) (-53.8445, 7.5731) (-54.1926, 7.5678) knots 0 0 0 0 1 1 1 1
  line L13 (-54.1926, 7.5678) -> (-56.2526, 7.5678)
  line L14 (-56.2526, 7.5678) -> (-56.2526, 5.5079)
  line L15 (-56.2526, 5.5079) -> (-54.1979, 5.5079)
  spline S15 degree 3 poles (-54.1979, 5.5079) (-53.8497, 5.5059) (-53.675, 5.3318) (-53.675, 4.985) knots 0 0 0 0 1 1 1 1
  spline S16 degree 3 poles (-53.675, 4.985) (-53.677, 4.6447) (-53.8478, 4.4733) (-54.1874, 4.47) knots 0 0 0 0 1 1 1 1
  line L16 (-54.1874, 4.47) -> (-56.7728, 4.47)
  spline S17 degree 3 poles (-56.7728, 4.47) (-57.1164, 4.47) (-57.2891, 4.6369) (-57.2905, 4.9719) knots 0 0 0 0 1 1 1 1
  line L17 (-57.2905, 4.9719) -> (-57.2905, 8.0881)
  spline S18 degree 3 poles (-57.2905, 8.0881) (-57.2891, 8.4297) (-57.1164, 8.6037) (-56.7728, 8.611) knots 0 0 0 0 1 1 1 1
  spline S19 degree 3 poles (-56.0056, 6.5274) (-56.0023, 6.8702) (-55.8315, 7.045) (-55.4932, 7.0502) knots 0 0 0 0 1 1 1 1
  line L18 (-55.4932, 7.0502) -> (-54.4528, 7.0502)
  spline S20 degree 3 poles (-54.4528, 7.0502) (-54.1079, 7.0463) (-53.9325, 6.8742) (-53.9273, 6.5326) knots 0 0 0 0 1 1 1 1
  spline S21 degree 3 poles (-53.9273, 6.5326) (-53.9345, 6.1871) (-54.1086, 6.015) (-54.4501, 6.015) knots 0 0 0 0 1 1 1 1
  line L19 (-54.4501, 6.015) -> (-55.4906, 6.015)
  spline S22 degree 3 poles (-55.4906, 6.015) (-55.8322, 6.013) (-56.0043, 6.1838) (-56.0056, 6.5274) knots 0 0 0 0 1 1 1 1
  spline S23 degree 3 poles (-52.6292, 8.6162) (-52.4578, 8.6162) (-52.3284, 8.5729) (-52.2404, 8.4875) knots 0 0 0 0 1 1 1 1
  spline S24 degree 3 poles (-52.2404, 8.4875) (-52.153, 8.4034) (-51.8462, 8.0434) (-51.3207, 7.4076) knots 0 0 0 0 1 1 1 1
  spline S25 degree 3 poles (-51.3207, 7.4076) (-50.7867, 8.0539) (-50.476, 8.4192) (-50.388, 8.5032) knots 0 0 0 0 1 1 1 1
  spline S26 degree 3 poles (-50.388, 8.5032) (-50.3006, 8.5873) (-50.1712, 8.6294) (-49.9991, 8.6294) knots 0 0 0 0 1 1 1 1
  spline S27 degree 3 poles (-49.9991, 8.6294) (-49.8309, 8.6294) (-49.7015, 8.5853) (-49.6102, 8.498) knots 0 0 0 0 1 1 1 1
  spline S28 degree 3 poles (-49.6102, 8.498) (-49.5196, 8.41) (-49.4762, 8.2799) (-49.4815, 8.1065) knots 0 0 0 0 1 1 1 1
  spline S29 degree 3 poles (-49.4815, 8.1065) (-49.4815, 7.9239) (-49.5728, 7.7531) (-49.7547, 7.5941) knots 0 0 0 0 1 1 1 1
  line L20 (-49.7547, 7.5941) -> (-50.8136, 6.3592)
  line L21 (-50.8136, 6.3592) -> (-50.8163, 4.985)
  spline S30 degree 3 poles (-50.8163, 4.985) (-50.8235, 4.6467) (-50.9969, 4.4753) (-51.3365, 4.47) knots 0 0 0 0 1 1 1 1
  spline S31 degree 3 poles (-51.3365, 4.47) (-51.6781, 4.4615) (-51.8489, 4.6382) (-51.8489, 5.0008) knots 0 0 0 0 1 1 1 1
  line L22 (-51.8489, 5.0008) -> (-51.8541, 6.3644)
  line L23 (-51.8541, 6.3644) -> (-52.8736, 7.5784)
  spline S32 degree 3 poles (-52.8736, 7.5784) (-53.0562, 7.7393) (-53.1468, 7.9107) (-53.1468, 8.0933) knots 0 0 0 0 1 1 1 1
  spline S33 degree 3 poles (-53.1468, 8.0933) (-53.1521, 8.2681) (-53.1101, 8.3988) (-53.0207, 8.4848) knots 0 0 0 0 1 1 1 1
  spline S34 degree 3 poles (-53.0207, 8.4848) (-52.9301, 8.5722) (-52.7994, 8.6162) (-52.6292, 8.6162) knots 0 0 0 0 1 1 1 1
  line L24 (-48.4962, 8.611) -> (-45.8792, 8.6057)
  spline S35 degree 3 poles (-45.8792, 8.6057) (-45.5574, 8.6004) (-45.3951, 8.4329) (-45.3931, 8.1039) knots 0 0 0 0 1 1 1 1
  spline S36 degree 3 poles (-45.3931, 8.1039) (-45.3931, 7.7518) (-45.5679, 7.5731) (-45.916, 7.5678) knots 0 0 0 0 1 1 1 1
  line L25 (-45.916, 7.5678) -> (-46.6885, 7.5678)
  line L26 (-46.6885, 7.5678) -> (-46.6859, 4.985)
  spline S37 degree 3 poles (-46.6859, 4.985) (-46.6898, 4.6447) (-46.8632, 4.4733) (-47.2061, 4.47) knots 0 0 0 0 1 1 1 1
  spline S38 degree 3 poles (-47.2061, 4.47) (-47.5516, 4.47) (-47.7237, 4.6369) (-47.7237, 4.9719) knots 0 0 0 0 1 1 1 1
  line L27 (-47.7237, 4.9719) -> (-47.7211, 7.5678)
  line L28 (-47.7211, 7.5678) -> (-48.4962, 7.5678)
  spline S39 degree 3 poles (-48.4962, 7.5678) (-48.8417, 7.5678) (-49.0138, 7.7413) (-49.0138, 8.0881) knots 0 0 0 0 1 1 1 1
  spline S40 degree 3 poles (-49.0138, 8.0881) (-49.0125, 8.4297) (-48.8398, 8.6037) (-48.4962, 8.611) knots 0 0 0 0 1 1 1 1
  spline S41 degree 3 poles (-44.3579, 4.4674) (-44.4459, 4.4674) (-44.5306, 4.4891) (-44.6127, 4.5331) knots 0 0 0 0 1 1 1 1
  spline S42 degree 3 poles (-44.6127, 4.5331) (-44.6955, 4.5764) (-44.7599, 4.6395) (-44.8072, 4.7223) knots 0 0 0 0 1 1 1 1
  spline S43 degree 3 poles (-44.8072, 4.7223) (-44.8531, 4.8063) (-44.8755, 4.8937) (-44.8755, 4.985) knots 0 0 0 0 1 1 1 1
  spline S44 degree 3 poles (-44.8755, 4.985) (-44.8755, 5.0743) (-44.618, 5.6366) (-44.103, 6.6719) knots 0 0 0 0 1 1 1 1
  spline S45 degree 3 poles (-44.103, 6.6719) (-43.5867, 7.7084) (-43.3062, 8.2681) (-43.2622, 8.3508) knots 0 0 0 0 1 1 1 1
  spline S46 degree 3 poles (-43.2622, 8.3508) (-43.2169, 8.4329) (-43.1532, 8.4967) (-43.0704, 8.5426) knots 0 0 0 0 1 1 1 1
  spline S47 degree 3 poles (-43.0704, 8.5426) (-42.9883, 8.588) (-42.9016, 8.611) (-42.8103, 8.611) knots 0 0 0 0 1 1 1 1
  spline S48 degree 3 poles (-42.8103, 8.611) (-42.7209, 8.611) (-42.6362, 8.588) (-42.5554, 8.5426) knots 0 0 0 0 1 1 1 1
  spline S49 degree 3 poles (-42.5554, 8.5426) (-42.4733, 8.4967) (-42.4096, 8.4329) (-42.3636, 8.3508) knots 0 0 0 0 1 1 1 1
  spline S50 degree 3 poles (-42.3636, 8.3508) (-42.3183, 8.2681) (-42.0365, 7.7084) (-41.5175, 6.6719) knots 0 0 0 0 1 1 1 1
  spline S51 degree 3 poles (-41.5175, 6.6719) (-40.9993, 5.6366) (-40.7398, 5.0743) (-40.7398, 4.985) knots 0 0 0 0 1 1 1 1
  spline S52 degree 3 poles (-40.7398, 4.985) (-40.7398, 4.8937) (-40.7634, 4.8063) (-40.8107, 4.7223) knots 0 0 0 0 1 1 1 1
  spline S53 degree 3 poles (-40.8107, 4.7223) (-40.8567, 4.6395) (-40.9211, 4.5764) (-41.0052, 4.5331) knots 0 0 0 0 1 1 1 1
  spline S54 degree 3 poles (-41.0052, 4.5331) (-41.0879, 4.4891) (-41.172, 4.4674) (-41.2574, 4.4674) knots 0 0 0 0 1 1 1 1
  line L29 (-41.2574, 4.4674) -> (-44.3579, 4.4674)
  line L30 (-42.1035, 5.5105) -> (-42.8103, 6.9661)
  line L31 (-42.8103, 6.9661) -> (-43.5223, 5.5105)
  line L32 (-43.5223, 5.5105) -> (-42.1035, 5.5105)
  spline S55 degree 3 poles (-35.8283, 8.6057) (-34.6216, 8.607) (-34.0173, 7.918) (-34.0153, 6.5379) knots 0 0 0 0 1 1 1 1
  spline S56 degree 3 poles (-34.0153, 6.5379) (-34.014, 6.1923) (-34.1861, 6.0209) (-34.5329, 6.0229) knots 0 0 0 0 1 1 1 1
  line L33 (-34.5329, 6.0229) -> (-36.6034, 6.0255)
  spline S57 degree 3 poles (-36.6034, 6.0255) (-36.6001, 5.6787) (-36.3426, 5.5039) (-35.8309, 5.5026) knots 0 0 0 0 1 1 1 1
  line L34 (-35.8309, 5.5026) -> (-34.5303, 5.5079)
  spline S58 degree 3 poles (-34.5303, 5.5079) (-34.1926, 5.5059) (-34.0205, 5.3325) (-34.0153, 4.9876) knots 0 0 0 0 1 1 1 1
  spline S59 degree 3 poles (-34.0153, 4.9876) (-34.0173, 4.6408) (-34.19, 4.4687) (-34.5329, 4.47) knots 0 0 0 0 1 1 1 1
  line L35 (-34.5329, 4.47) -> (-35.823, 4.47)
  spline S60 degree 3 poles (-35.823, 4.47) (-37.0336, 4.4713) (-37.6399, 5.1617) (-37.6412, 6.5405) knots 0 0 0 0 1 1 1 1
  spline S61 degree 3 poles (-37.6412, 6.5405) (-37.6399, 6.8821) (-37.4672, 7.0535) (-37.1236, 7.0555) knots 0 0 0 0 1 1 1 1
  line L36 (-37.1236, 7.0555) -> (-35.0532, 7.0529)
  spline S62 degree 3 poles (-35.0532, 7.0529) (-35.0532, 7.3977) (-35.308, 7.5692) (-35.8178, 7.5678) knots 0 0 0 0 1 1 1 1
  line L37 (-35.8178, 7.5678) -> (-37.1184, 7.5678)
  spline S63 degree 3 poles (-37.1184, 7.5678) (-37.4599, 7.5764) (-37.6347, 7.7505) (-37.6412, 8.0907) knots 0 0 0 0 1 1 1 1
  spline S64 degree 3 poles (-37.6412, 8.0907) (-37.6327, 8.4356) (-37.4586, 8.607) (-37.1184, 8.6057) knots 0 0 0 0 1 1 1 1
  line L38 (-37.1184, 8.6057) -> (-35.8283, 8.6057)
  spline S65 degree 3 poles (-31.4351, 8.6057) (-31.0883, 8.6057) (-30.7506, 8.5164) (-30.4209, 8.3377) knots 0 0 0 0 1 1 1 1
  spline S66 degree 3 poles (-30.4209, 8.3377) (-30.0898, 8.159) (-29.831, 7.9028) (-29.6431, 7.5705) knots 0 0 0 0 1 1 1 1
  spline S67 degree 3 poles (-29.6431, 7.5705) (-29.4559, 7.2394) (-29.362, 6.8939) (-29.362, 6.5352) knots 0 0 0 0 1 1 1 1
  spline S68 degree 3 poles (-29.362, 6.5352) (-29.362, 6.1759) (-29.4533, 5.8317) (-29.6353, 5.5026) knots 0 0 0 0 1 1 1 1
  spline S69 degree 3 poles (-29.6353, 5.5026) (-29.8179, 5.1748) (-30.0734, 4.92) (-30.4025, 4.738) knots 0 0 0 0 1 1 1 1
  spline S70 degree 3 poles (-30.4025, 4.738) (-30.7322, 4.5554) (-31.0764, 4.4648) (-31.4351, 4.4648) knots 0 0 0 0 1 1 1 1
  spline S71 degree 3 poles (-31.4351, 4.4648) (-31.7924, 4.4648) (-32.136, 4.5554) (-32.4651, 4.738) knots 0 0 0 0 1 1 1 1
  spline S72 degree 3 poles (-32.4651, 4.738) (-32.7948, 4.92) (-33.0503, 5.1748) (-33.2323, 5.5026) knots 0 0 0 0 1 1 1 1
  spline S73 degree 3 poles (-33.2323, 5.5026) (-33.4149, 5.8317) (-33.5056, 6.1759) (-33.5056, 6.5352) knots 0 0 0 0 1 1 1 1
  spline S74 degree 3 poles (-33.5056, 6.5352) (-33.5056, 6.8939) (-33.4136, 7.2394) (-33.2297, 7.5705) knots 0 0 0 0 1 1 1 1
  spline S75 degree 3 poles (-33.2297, 7.5705) (-33.0444, 7.9028) (-32.7869, 8.159) (-32.4572, 8.3377) knots 0 0 0 0 1 1 1 1
  spline S76 degree 3 poles (-32.4572, 8.3377) (-32.1261, 8.5164) (-31.7859, 8.6057) (-31.4351, 8.6057) knots 0 0 0 0 1 1 1 1
  spline S77 degree 3 poles (-31.4325, 7.5757) (-31.6078, 7.5757) (-31.778, 7.5311) (-31.9422, 7.4417) knots 0 0 0 0 1 1 1 1
  spline S78 degree 3 poles (-31.9422, 7.4417) (-32.1071, 7.3537) (-32.2358, 7.2269) (-32.3284, 7.0607) knots 0 0 0 0 1 1 1 1
  spline S79 degree 3 poles (-32.3284, 7.0607) (-32.4217, 6.8939) (-32.4677, 6.7205) (-32.4677, 6.5405) knots 0 0 0 0 1 1 1 1
  spline S80 degree 3 poles (-32.4677, 6.5405) (-32.4677, 6.3598) (-32.4224, 6.1871) (-32.3311, 6.0229) knots 0 0 0 0 1 1 1 1
  spline S81 degree 3 poles (-32.3311, 6.0229) (-32.2404, 5.86) (-32.1123, 5.7325) (-31.9474, 5.6419) knots 0 0 0 0 1 1 1 1
  spline S82 degree 3 poles (-31.9474, 5.6419) (-31.7832, 5.5506) (-31.6111, 5.5053) (-31.4325, 5.5053) knots 0 0 0 0 1 1 1 1
  spline S83 degree 3 poles (-31.4325, 5.5053) (-31.2525, 5.5053) (-31.0797, 5.5506) (-30.9148, 5.6419) knots 0 0 0 0 1 1 1 1
  spline S84 degree 3 poles (-30.9148, 5.6419) (-30.7506, 5.7325) (-30.6225, 5.86) (-30.5312, 6.0229) knots 0 0 0 0 1 1 1 1
  spline S85 degree 3 poles (-30.5312, 6.0229) (-30.4406, 6.1871) (-30.3946, 6.3598) (-30.3946, 6.5405) knots 0 0 0 0 1 1 1 1
  spline S86 degree 3 poles (-30.3946, 6.5405) (-30.3946, 6.7205) (-30.4412, 6.8939) (-30.5339, 7.0607) knots 0 0 0 0 1 1 1 1
  spline S87 degree 3 poles (-30.5339, 7.0607) (-30.6271, 7.2269) (-30.7565, 7.3537) (-30.9227, 7.4417) knots 0 0 0 0 1 1 1 1
  spline S88 degree 3 poles (-30.9227, 7.4417) (-31.0876, 7.5311) (-31.2577, 7.5757) (-31.4325, 7.5757) knots 0 0 0 0 1 1 1 1
  spline S89 degree 3 poles (-31.4351, 7.045) (-31.3497, 7.045) (-31.2663, 7.022) (-31.1855, 6.9767) knots 0 0 0 0 1 1 1 1
  spline S90 degree 3 poles (-31.1855, 6.9767) (-31.1034, 6.9326) (-31.0396, 6.8696) (-30.9937, 6.7875) knots 0 0 0 0 1 1 1 1
  spline S91 degree 3 poles (-30.9937, 6.7875) (-30.9464, 6.7067) (-30.9227, 6.6206) (-30.9227, 6.53) knots 0 0 0 0 1 1 1 1
  spline S92 degree 3 poles (-30.9227, 6.53) (-30.9227, 6.4406) (-30.9457, 6.3546) (-30.991, 6.2725) knots 0 0 0 0 1 1 1 1
  spline S93 degree 3 poles (-30.991, 6.2725) (-31.037, 6.1917) (-31.1001, 6.1286) (-31.1802, 6.0833) knots 0 0 0 0 1 1 1 1
  spline S94 degree 3 poles (-31.1802, 6.0833) (-31.261, 6.0393) (-31.3458, 6.0176) (-31.4351, 6.0176) knots 0 0 0 0 1 1 1 1
  spline S95 degree 3 poles (-31.4351, 6.0176) (-31.5264, 6.0176) (-31.6131, 6.0393) (-31.6952, 6.0833) knots 0 0 0 0 1 1 1 1
  spline S96 degree 3 poles (-31.6952, 6.0833) (-31.776, 6.1286) (-31.8391, 6.1917) (-31.8844, 6.2725) knots 0 0 0 0 1 1 1 1
  spline S97 degree 3 poles (-31.8844, 6.2725) (-31.9284, 6.3546) (-31.9501, 6.4406) (-31.9501, 6.53) knots 0 0 0 0 1 1 1 1
  spline S98 degree 3 poles (-31.9501, 6.53) (-31.9501, 6.6206) (-31.9277, 6.7067) (-31.8818, 6.7875) knots 0 0 0 0 1 1 1 1
  spline S99 degree 3 poles (-31.8818, 6.7875) (-31.8364, 6.8696) (-31.7734, 6.9326) (-31.6926, 6.9767) knots 0 0 0 0 1 1 1 1
  spline S100 degree 3 poles (-31.6926, 6.9767) (-31.6105, 7.022) (-31.5244, 7.045) (-31.4351, 7.045) knots 0 0 0 0 1 1 1 1
  spline S101 degree 3 poles (-26.7769, 8.6057) (-26.4301, 8.6057) (-26.0924, 8.5164) (-25.7627, 8.3377) knots 0 0 0 0 1 1 1 1
  spline S102 degree 3 poles (-25.7627, 8.3377) (-25.4316, 8.159) (-25.1728, 7.9028) (-24.9849, 7.5705) knots 0 0 0 0 1 1 1 1
  spline S103 degree 3 poles (-24.9849, 7.5705) (-24.7977, 7.2394) (-24.7038, 6.8939) (-24.7038, 6.5352) knots 0 0 0 0 1 1 1 1
  spline S104 degree 3 poles (-24.7038, 6.5352) (-24.7038, 6.1759) (-24.7951, 5.8317) (-24.9771, 5.5026) knots 0 0 0 0 1 1 1 1
  spline S105 degree 3 poles (-24.9771, 5.5026) (-25.1597, 5.1748) (-25.4152, 4.92) (-25.7443, 4.738) knots 0 0 0 0 1 1 1 1
  spline S106 degree 3 poles (-25.7443, 4.738) (-26.074, 4.5554) (-26.4182, 4.4648) (-26.7769, 4.4648) knots 0 0 0 0 1 1 1 1
  spline S107 degree 3 poles (-26.7769, 4.4648) (-27.1342, 4.4648) (-27.4778, 4.5554) (-27.8069, 4.738) knots 0 0 0 0 1 1 1 1
  spline S108 degree 3 poles (-27.8069, 4.738) (-28.1366, 4.92) (-28.3922, 5.1748) (-28.5741, 5.5026) knots 0 0 0 0 1 1 1 1
  spline S109 degree 3 poles (-28.5741, 5.5026) (-28.7567, 5.8317) (-28.8474, 6.1759) (-28.8474, 6.5352) knots 0 0 0 0 1 1 1 1
  spline S110 degree 3 poles (-28.8474, 6.5352) (-28.8474, 6.8939) (-28.7554, 7.2394) (-28.5715, 7.5705) knots 0 0 0 0 1 1 1 1
  spline S111 degree 3 poles (-28.5715, 7.5705) (-28.3862, 7.9028) (-28.1288, 8.159) (-27.799, 8.3377) knots 0 0 0 0 1 1 1 1
  spline S112 degree 3 poles (-27.799, 8.3377) (-27.4679, 8.5164) (-27.1277, 8.6057) (-26.7769, 8.6057) knots 0 0 0 0 1 1 1 1
  spline S113 degree 3 poles (-26.7743, 7.5757) (-26.9497, 7.5757) (-27.1198, 7.5311) (-27.284, 7.4417) knots 0 0 0 0 1 1 1 1
  spline S114 degree 3 poles (-27.284, 7.4417) (-27.4489, 7.3537) (-27.5776, 7.2269) (-27.6703, 7.0607) knots 0 0 0 0 1 1 1 1
  spline S115 degree 3 poles (-27.6703, 7.0607) (-27.7635, 6.8939) (-27.8095, 6.7205) (-27.8095, 6.5405) knots 0 0 0 0 1 1 1 1
  spline S116 degree 3 poles (-27.8095, 6.5405) (-27.8095, 6.3598) (-27.7642, 6.1871) (-27.6729, 6.0229) knots 0 0 0 0 1 1 1 1
  spline S117 degree 3 poles (-27.6729, 6.0229) (-27.5822, 5.86) (-27.4541, 5.7325) (-27.2893, 5.6419) knots 0 0 0 0 1 1 1 1
  spline S118 degree 3 poles (-27.2893, 5.6419) (-27.125, 5.5506) (-26.9529, 5.5053) (-26.7743, 5.5053) knots 0 0 0 0 1 1 1 1
  spline S119 degree 3 poles (-26.7743, 5.5053) (-26.5943, 5.5053) (-26.4215, 5.5506) (-26.2567, 5.6419) knots 0 0 0 0 1 1 1 1
  spline S120 degree 3 poles (-26.2567, 5.6419) (-26.0924, 5.7325) (-25.9643, 5.86) (-25.873, 6.0229) knots 0 0 0 0 1 1 1 1
  spline S121 degree 3 poles (-25.873, 6.0229) (-25.7824, 6.1871) (-25.7364, 6.3598) (-25.7364, 6.5405) knots 0 0 0 0 1 1 1 1
  spline S122 degree 3 poles (-25.7364, 6.5405) (-25.7364, 6.7205) (-25.7831, 6.8939) (-25.8757, 7.0607) knots 0 0 0 0 1 1 1 1
  spline S123 degree 3 poles (-25.8757, 7.0607) (-25.9689, 7.2269) (-26.0984, 7.3537) (-26.2645, 7.4417) knots 0 0 0 0 1 1 1 1
  spline S124 degree 3 poles (-26.2645, 7.4417) (-26.4294, 7.5311) (-26.5995, 7.5757) (-26.7743, 7.5757) knots 0 0 0 0 1 1 1 1
  spline S125 degree 3 poles (-26.7769, 7.045) (-26.6915, 7.045) (-26.6081, 7.022) (-26.5273, 6.9767) knots 0 0 0 0 1 1 1 1
  spline S126 degree 3 poles (-26.5273, 6.9767) (-26.4452, 6.9326) (-26.3815, 6.8696) (-26.3355, 6.7875) knots 0 0 0 0 1 1 1 1
  spline S127 degree 3 poles (-26.3355, 6.7875) (-26.2882, 6.7067) (-26.2645, 6.6206) (-26.2645, 6.53) knots 0 0 0 0 1 1 1 1
  spline S128 degree 3 poles (-26.2645, 6.53) (-26.2645, 6.4406) (-26.2875, 6.3546) (-26.3329, 6.2725) knots 0 0 0 0 1 1 1 1
  spline S129 degree 3 poles (-26.3329, 6.2725) (-26.3788, 6.1917) (-26.4419, 6.1286) (-26.522, 6.0833) knots 0 0 0 0 1 1 1 1
  spline S130 degree 3 poles (-26.522, 6.0833) (-26.6028, 6.0393) (-26.6876, 6.0176) (-26.7769, 6.0176) knots 0 0 0 0 1 1 1 1
  spline S131 degree 3 poles (-26.7769, 6.0176) (-26.8682, 6.0176) (-26.9549, 6.0393) (-27.037, 6.0833) knots 0 0 0 0 1 1 1 1
  spline S132 degree 3 poles (-27.037, 6.0833) (-27.1178, 6.1286) (-27.1809, 6.1917) (-27.2262, 6.2725) knots 0 0 0 0 1 1 1 1
  spline S133 degree 3 poles (-27.2262, 6.2725) (-27.2702, 6.3546) (-27.2919, 6.4406) (-27.2919, 6.53) knots 0 0 0 0 1 1 1 1
  spline S134 degree 3 poles (-27.2919, 6.53) (-27.2919, 6.6206) (-27.2696, 6.7067) (-27.2236, 6.7875) knots 0 0 0 0 1 1 1 1
  spline S135 degree 3 poles (-27.2236, 6.7875) (-27.1783, 6.8696) (-27.1152, 6.9326) (-27.0344, 6.9767) knots 0 0 0 0 1 1 1 1
  spline S136 degree 3 poles (-27.0344, 6.9767) (-26.9523, 7.022) (-26.8662, 7.045) (-26.7769, 7.045) knots 0 0 0 0 1 1 1 1
  spline S137 degree 3 poles (-22.1187, 8.6057) (-21.7719, 8.6057) (-21.4343, 8.5164) (-21.1045, 8.3377) knots 0 0 0 0 1 1 1 1
  spline S138 degree 3 poles (-21.1045, 8.3377) (-20.7734, 8.159) (-20.5146, 7.9028) (-20.3268, 7.5705) knots 0 0 0 0 1 1 1 1
  spline S139 degree 3 poles (-20.3268, 7.5705) (-20.1396, 7.2394) (-20.0456, 6.8939) (-20.0456, 6.5352) knots 0 0 0 0 1 1 1 1
  spline S140 degree 3 poles (-20.0456, 6.5352) (-20.0456, 6.1759) (-20.1369, 5.8317) (-20.3189, 5.5026) knots 0 0 0 0 1 1 1 1
  spline S141 degree 3 poles (-20.3189, 5.5026) (-20.5015, 5.1748) (-20.757, 4.92) (-21.0861, 4.738) knots 0 0 0 0 1 1 1 1
  spline S142 degree 3 poles (-21.0861, 4.738) (-21.4159, 4.5554) (-21.7601, 4.4648) (-22.1187, 4.4648) knots 0 0 0 0 1 1 1 1
  spline S143 degree 3 poles (-22.1187, 4.4648) (-22.4761, 4.4648) (-22.8196, 4.5554) (-23.1487, 4.738) knots 0 0 0 0 1 1 1 1
  spline S144 degree 3 poles (-23.1487, 4.738) (-23.4784, 4.92) (-23.734, 5.1748) (-23.9159, 5.5026) knots 0 0 0 0 1 1 1 1
  spline S145 degree 3 poles (-23.9159, 5.5026) (-24.0985, 5.8317) (-24.1892, 6.1759) (-24.1892, 6.5352) knots 0 0 0 0 1 1 1 1
  spline S146 degree 3 poles (-24.1892, 6.5352) (-24.1892, 6.8939) (-24.0972, 7.2394) (-23.9133, 7.5705) knots 0 0 0 0 1 1 1 1
  spline S147 degree 3 poles (-23.9133, 7.5705) (-23.7281, 7.9028) (-23.4706, 8.159) (-23.1408, 8.3377) knots 0 0 0 0 1 1 1 1
  spline S148 degree 3 poles (-23.1408, 8.3377) (-22.8097, 8.5164) (-22.4695, 8.6057) (-22.1187, 8.6057) knots 0 0 0 0 1 1 1 1
  spline S149 degree 3 poles (-22.1161, 7.5757) (-22.2915, 7.5757) (-22.4616, 7.5311) (-22.6258, 7.4417) knots 0 0 0 0 1 1 1 1
  spline S150 degree 3 poles (-22.6258, 7.4417) (-22.7907, 7.3537) (-22.9194, 7.2269) (-23.0121, 7.0607) knots 0 0 0 0 1 1 1 1
  spline S151 degree 3 poles (-23.0121, 7.0607) (-23.1053, 6.8939) (-23.1513, 6.7205) (-23.1513, 6.5405) knots 0 0 0 0 1 1 1 1
  spline S152 degree 3 poles (-23.1513, 6.5405) (-23.1513, 6.3598) (-23.106, 6.1871) (-23.0147, 6.0229) knots 0 0 0 0 1 1 1 1
  spline S153 degree 3 poles (-23.0147, 6.0229) (-22.924, 5.86) (-22.796, 5.7325) (-22.6311, 5.6419) knots 0 0 0 0 1 1 1 1
  spline S154 degree 3 poles (-22.6311, 5.6419) (-22.4669, 5.5506) (-22.2948, 5.5053) (-22.1161, 5.5053) knots 0 0 0 0 1 1 1 1
  spline S155 degree 3 poles (-22.1161, 5.5053) (-21.9361, 5.5053) (-21.7633, 5.5506) (-21.5985, 5.6419) knots 0 0 0 0 1 1 1 1
  spline S156 degree 3 poles (-21.5985, 5.6419) (-21.4343, 5.7325) (-21.3062, 5.86) (-21.2149, 6.0229) knots 0 0 0 0 1 1 1 1
  spline S157 degree 3 poles (-21.2149, 6.0229) (-21.1242, 6.1871) (-21.0782, 6.3598) (-21.0782, 6.5405) knots 0 0 0 0 1 1 1 1
  spline S158 degree 3 poles (-21.0782, 6.5405) (-21.0782, 6.7205) (-21.1249, 6.8939) (-21.2175, 7.0607) knots 0 0 0 0 1 1 1 1
  spline S159 degree 3 poles (-21.2175, 7.0607) (-21.3108, 7.2269) (-21.4402, 7.3537) (-21.6064, 7.4417) knots 0 0 0 0 1 1 1 1
  spline S160 degree 3 poles (-21.6064, 7.4417) (-21.7712, 7.5311) (-21.9414, 7.5757) (-22.1161, 7.5757) knots 0 0 0 0 1 1 1 1
  spline S161 degree 3 poles (-22.1187, 7.045) (-22.0333, 7.045) (-21.9499, 7.022) (-21.8691, 6.9767) knots 0 0 0 0 1 1 1 1
  spline S162 degree 3 poles (-21.8691, 6.9767) (-21.787, 6.9326) (-21.7233, 6.8696) (-21.6773, 6.7875) knots 0 0 0 0 1 1 1 1
  spline S163 degree 3 poles (-21.6773, 6.7875) (-21.63, 6.7067) (-21.6064, 6.6206) (-21.6064, 6.53) knots 0 0 0 0 1 1 1 1
  spline S164 degree 3 poles (-21.6064, 6.53) (-21.6064, 6.4406) (-21.6293, 6.3546) (-21.6747, 6.2725) knots 0 0 0 0 1 1 1 1
  spline S165 degree 3 poles (-21.6747, 6.2725) (-21.7207, 6.1917) (-21.7837, 6.1286) (-21.8638, 6.0833) knots 0 0 0 0 1 1 1 1
  spline S166 degree 3 poles (-21.8638, 6.0833) (-21.9446, 6.0393) (-22.0294, 6.0176) (-22.1187, 6.0176) knots 0 0 0 0 1 1 1 1
  spline S167 degree 3 poles (-22.1187, 6.0176) (-22.21, 6.0176) (-22.2967, 6.0393) (-22.3788, 6.0833) knots 0 0 0 0 1 1 1 1
  spline S168 degree 3 poles (-22.3788, 6.0833) (-22.4596, 6.1286) (-22.5227, 6.1917) (-22.568, 6.2725) knots 0 0 0 0 1 1 1 1
  spline S169 degree 3 poles (-22.568, 6.2725) (-22.612, 6.3546) (-22.6337, 6.4406) (-22.6337, 6.53) knots 0 0 0 0 1 1 1 1
  spline S170 degree 3 poles (-22.6337, 6.53) (-22.6337, 6.6206) (-22.6114, 6.7067) (-22.5654, 6.7875) knots 0 0 0 0 1 1 1 1